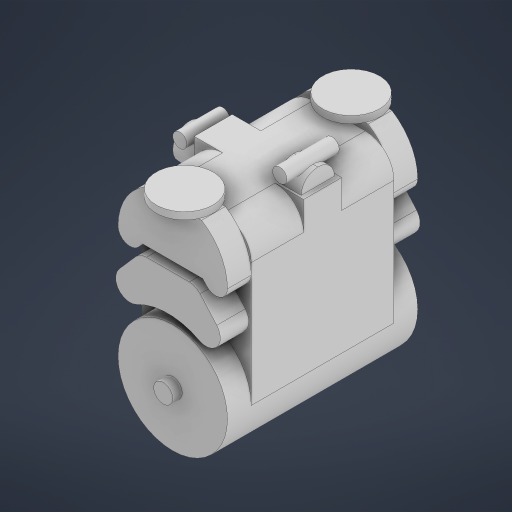
# Autodesk Inventor part: cylinder
Saved by Autodesk Inventor 2023 (Build 270158000, 158)
## iProperties
Created: 2023-09-11
Part Number: cylinder
Material: Generic
Document SubType Name: Modeling
Designer: Peter
Density: 1 g/cm^3
Appearance: Default
Author: Peter
Autodesk Inventor part; units mm, degrees
ref_plane "YZ Plane" through (0, 0, 0) normal (1, 0, 0) x (0, 1, 0)
ref_plane "XZ Plane" through (0, 0, 0) normal (0, 1, 0) x (-1, 0, 0)
ref_plane "XY Plane" through (0, 0, 0) normal (0, 0, 1) x (1, 0, 0)
sketch "Sketch1" plane through (0, 0, 0) normal (0, 0, 1) x (1, 0, 0)
  arc A0 (-292.1, 0) -> (292.1, 0) centre (0, 0) ccw
  arc A1 (292.1, 660.4) -> (139.7, 812.8) centre (139.7, 660.4) ccw
  arc A2 (-139.7, 812.8) -> (-292.1, 660.4) centre (-139.7, 660.4) ccw
  line L0 (-139.7, 812.8) -> (139.7, 812.8)
  line L1 (0, -519.3926) -> (0, 1071.6557) construction
  line L2 (-292.1, 660.4) -> (-292.1, 0)
  line L3 (292.1, 660.4) -> (292.1, 0)
  point P0 (0, 812.8)
  dimension "d0" = 584.2
  dimension "d1" = 304.8
  dimension "d2" = 304.8
  dimension "d3" = 812.8
  constraints: 6 end point, 6 point on circle, 5 tangent, 3 centre point, 2 vertical, 1 coincident, 1 horizontal, 1 midpoint, 1 point on line
  measures "d0" diameter of A0
  measures "d1" diameter of A2
  measures "d2" diameter of A1
  measures "d3" distance from line of point (0, 0) L0
extrude "Extrusion1" add sketch "Sketch1" along normal blind 381
sketch "Sketch2" plane through (0, 0, 381) normal (0, 0, 1) x (1, 0, 0)
  circle A0 centre (0, 0) radius 292.1
  arc A1 (-292.1, 0) -> (292.1, 0) centre (0, 0) ccw construction
  dimension "d9" = 584.2
  dimension "d10" = 584.2
  constraints: 1 centre point, 1 coincident
  measures "d9" diameter of A1
  measures "d10" diameter of A0
extrude "Extrusion2" add sketch "Sketch2" along normal blind 127
sketch "Sketch4" plane through (0, 0, 381) normal (0, 0, 1) x (1, 0, 0)
  arc A0 (167.3412, 313.7647) -> (-167.3412, 313.7647) centre (0, 0) ccw
  line L0 (-260.5463, 431.1781) -> (-171.6463, 532.7781)
  line L1 (-114.3, 558.8) -> (114.3, 558.8)
  line L2 (171.6463, 532.7781) -> (260.5463, 431.1781)
  arc A1 (-114.3, 558.8) -> (-171.6463, 532.7781) centre (-114.3, 482.6) ccw
  arc A2 (171.6463, 532.7781) -> (114.3, 558.8) centre (114.3, 482.6) ccw
  arc A3 (167.3412, 313.7647) -> (260.5463, 431.1781) centre (203.2, 381) ccw
  arc A4 (-260.5463, 431.1781) -> (-167.3412, 313.7647) centre (-203.2, 381) ccw
  line L3 (-114.3, 482.6) -> (114.3, 482.6) construction
  line L4 (203.2, 381) -> (-203.2, 381) construction
  line L5 (0, -513.08) -> (0, 1033.78) construction
  point P0 (0, 482.6)
  dimension "d22" = 355.6
  dimension "d23" = 76.2
  dimension "d24" = 406.4
  dimension "d25" = 558.8
  dimension "d26" = 228.6
  constraints: 10 end point, 10 point on circle, 8 tangent, 5 centre point, 3 equal radius, 3 horizontal, 1 coincident, 1 midpoint, 1 point on line
  measures "d22" radius of A0
  measures "d23" radius of A1
  measures "d24" distance of L4.start L4.end
  measures "d25" distance from line of point (0, 0) L1
  measures "d26" distance of L3.start L3.end
extrude "Extrusion4" add sketch "Sketch4" along normal blind 152.4
sketch "Sketch5" plane through (0, 0, 381) normal (0, 0, 1) x (1, 0, 0)
  arc A0 (-292.1, 602.691) -> (-180.8114, 560.876) centre (-228.6, 602.691) ccw
  arc A1 (180.8114, 560.876) -> (292.1, 602.691) centre (228.6, 602.691) ccw
  line L0 (228.6, 602.691) -> (-228.6, 602.691) construction
  line L1 (0, -524.2834) -> (0, 1101.0005) construction
  line L2 (-180.8114, 560.876) -> (-160.4029, 584.2)
  line L3 (-160.4029, 584.2) -> (160.4029, 584.2)
  line L4 (160.4029, 584.2) -> (180.8114, 560.876)
  line L5 (-171.6463, 532.7781) -> (-260.5463, 431.1781) projected
  line L6 (114.3, 558.8) -> (-114.3, 558.8) projected
  arc A2 (-153.9958, 850.9) -> (-292.1, 602.691) centre (0, 602.691) ccw
  arc A3 (292.1, 602.691) -> (153.9958, 850.9) centre (0, 602.691) ccw
  line L7 (-153.9958, 850.9) -> (153.9958, 850.9)
  line L8 (139.7, 812.8) -> (-139.7, 812.8) construction
  line L9 (-292.1, 660.4) -> (-292.1, 0) construction
  point P0 (0, 0)
  dimension "d29" = 127
  dimension "d31" = 25.4
  dimension "d32" = 25.4
  dimension "d35" = 266.7
  constraints: 10 end point, 10 point on circle, 4 centre point, 4 tangent, 2 coincident, 2 horizontal, 2 parallel, 2 point on line, 1 concentric, 1 horizontal alignment, 1 midpoint
  measures "d29" diameter of A0
  measures "d31" distance between parallel lines of L2 L5
  measures "d32" distance between parallel lines of L6 L3
  measures "d35" distance between parallel lines of L3 L7
extrude "Extrusion5" add sketch "Sketch5" along normal blind 127
sketch "Sketch6" plane through (292.1, 0, 0) normal (1, 0, 0) x (0, 0, -1)
  line L0 (0, 812.8) -> (-101.6, 812.8)
  line L1 (-101.6, 812.8) -> (-101.6, 355.6)
  line L2 (0, 254) -> (0, 812.8)
  arc A0 (-101.6, 355.6) -> (0, 254) centre (0, 355.6) ccw
  line L3 (0, 0) -> (0, 660.4) projected
  line L4 (0, -530.86) -> (0, 1140.46) construction
  line L5 (0, 812.8) -> (-381, 812.8) construction
  line L6 (0, 812.8) -> (-381, 812.8) construction
  point P0 (-50.8, 812.8)
  point P1 (0, 901.7)
  dimension "d38" = 101.6
  dimension "d39" = 558.8
  constraints: 7 end point, 4 point on line, 2 point on circle, 1 centre point, 1 horizontal, 1 midpoint, 1 parallel, 1 perpendicular, 1 tangent
  measures "d38" distance between parallel lines of L2 L1
  measures "d39" vertical distance of L2.start point (-50.8, 812.8)
extrude "Extrusion6" add sketch "Sketch6" against normal up to surface (584.2 mm away)
sketch "Sketch7" plane through (-153.9958, 850.9, 381) normal (0, 1, 0) x (1, 0, 0)
  line L0 (307.9916, 0) -> (307.9916, -127) construction
  line L1 (-17.6505, 0) -> (-17.6505, -152.4) construction
  line L2 (-17.6505, -63.5) -> (307.9916, -63.5) construction
  line L3 (153.9958, 500.38) -> (153.9958, -335.28) construction
  circle A0 centre (153.9958, -63.5) radius 152.4
  point P0 (153.9958, 381)
  dimension "d43" = 304.8
  constraints: 3 point on line, 2 end point, 1 centre point, 1 coincident, 1 horizontal, 1 midpoint
  measures "d43" diameter of A0
extrude "Extrusion7" add sketch "Sketch7" along normal blind 38.1
sketch "Sketch8" plane through (0, 0, 508) normal (0, 0, 1) x (1, 0, 0)
  circle A0 centre (0, 0) radius 50.8
  dimension "d46" = 101.6
  constraints: 1 centre point, 1 coincident
  measures "d46" diameter of A0
extrude "Extrusion8" add sketch "Sketch8" along normal blind 50.8
ref_plane "Work Plane2" through (266.7, 0, 0) normal (1, 0, 0) x (0, 0, -1)
sketch "Sketch10" plane through (266.7, 0, 0) normal (1, 0, 0) x (0, 0, -1)
  arc A0 (0, 899.6714) -> (-88.9, 812.8) centre (-2.0054, 812.8) ccw
  line L0 (-88.9, 812.8) -> (0, 812.8)
  line L1 (0, 812.8) -> (0, 899.6714)
  point P0 (0, 0)
  point P1 (-101.6, 812.8)
  dimension "d57" = 0
  dimension "d58" = 12.7
  constraints: 4 end point, 2 point on circle, 1 centre point, 1 horizontal, 1 vertical
  measures "d57" vertical distance of A0.centre L0.end
  measures "d58" distance of L0.start point (-101.6, 812.8)
extrude "Extrusion9" add sketch "Sketch10" against normal blind 127
mirror "Mirror3" about plane through (0, 0, 0) normal (0, 0, 1)
sketch "Sketch11" plane through (0, 0, 0) normal (0, 0, 1) x (1, 0, 0)
  line L0 (266.7, 899.6714) -> (139.7, 899.6714) construction
  circle A0 centre (203.2, 899.6714) radius 38.1
  point P0 (0, 0)
  dimension "d59" = 76.2
  constraints: 1 centre point, 1 coincident, 1 midpoint
  measures "d59" diameter of A0
extrude "Extrusion10" add sketch "Sketch11" along normal mid plane 279.4
sketch "Sketch12" plane through (-292.1, 0, 381) normal (-1, 0, 0) x (0, 0, 1)
  circle A0 centre (-381, 680.5884) radius 88.9
  line L0 (-762, 0) -> (0, 0) construction
  line L1 (-279.4, 812.8) -> (-279.4, 660.4) construction
  point P0 (-381, 0)
  point P1 (-381, 0)
  point P2 (-292.1, 680.5884)
  dimension "d60" = 0
  dimension "d64" = 12.7
  constraints: 1 horizontal alignment, 1 midpoint, 2 other
  measures "d60" horizontal distance of point (-381, 0) point (-381, 680.588)
  measures "d64" distance from line of point (-292.1, 680.588) L1
extrude "Extrusion11" add sketch "Sketch12" along normal blind 127
sketch "Sketch13" plane through (0, 0, 0) normal (0, 0, 1) x (1, 0, 0)
  line L0 (-292.1, 769.4884) -> (-419.1, 769.4884) construction
  circle A0 centre (-355.6, 769.4884) radius 38.1
  point P0 (0, 0)
  dimension "d65" = 76.2
  constraints: 1 centre point, 1 coincident, 1 midpoint
  measures "d65" diameter of A0
extrude "Extrusion12" add sketch "Sketch13" along normal mid plane 228.6
equation "\"d2\" = d1"
equation "\"d10\" = d9"
body "Solid1"
